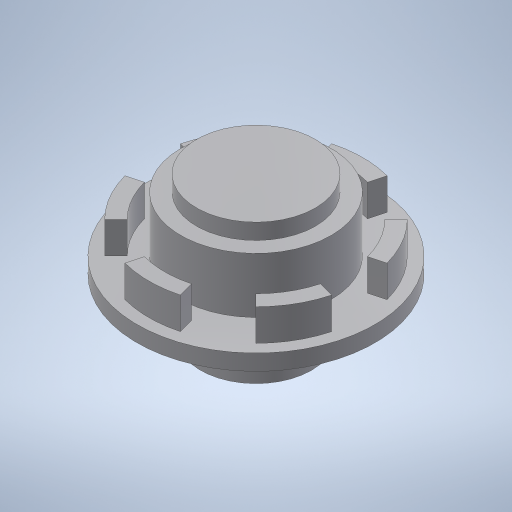
# Autodesk Inventor part: Bisagra final
Saved by Autodesk Inventor 2023.1 (Build 271208000, 208)
## iProperties
Created: 2022-10-06
Part Number: Bisagra final
Material: Generic
Document SubType Name: Modeling
Designer: User
Density: 1 g/cm^3
Appearance: Smooth - White
Author: User
Autodesk Inventor part; units mm, degrees
ref_plane "YZ Plane" through (0, 0, 0) normal (1, 0, 0) x (0, 1, 0)
ref_plane "XZ Plane" through (0, 0, 0) normal (0, 1, 0) x (-1, 0, 0)
ref_plane "XY Plane" through (0, 0, 0) normal (0, 0, 1) x (1, 0, 0)
sketch "Sketch1" plane through (0, 0, 0) normal (0, 1, 0) x (-1, 0, 0)
  circle A0 centre (0, 0) radius 15
  dimension "d0" = 30
  constraints: 1 centre point, 1 coincident
  measures "d0" diameter of A0
extrude "Extrusion1" add sketch "Sketch1" along normal blind 2
sketch "Sketch2" plane through (0, 2, 0) normal (0, 1, 0) x (1, 0, 0)
  circle A0 centre (0, 0) radius 15 projected
  circle A1 centre (0, 0) radius 13.5
  circle A2 centre (0, 0) radius 11.5
  line L0 (11.1081, 2.9764) -> (13.04, 3.4941)
  line L1 (0, 0) -> (13.5, 0) construction
  line L2 (11.1081, -2.9764) -> (13.04, -3.4941)
  line L3 (0, 0) -> (13.5, 0) construction
  line L4 (8.1317, 8.1317) -> (9.5459, 9.5459)
  line L5 (0, 0) -> (13.5, 0) construction
  line L6 (2.9764, 11.1081) -> (3.4941, 13.04)
  line L7 (0, 0) -> (13.5, 0) construction
  line L8 (-2.9764, 11.1081) -> (-3.4941, 13.04)
  circle A3 centre (0, 0) radius 15 projected
  line L9 (-8.1317, 8.1317) -> (-9.5459, 9.5459)
  line L10 (0, 0) -> (13.5, 0) construction
  line L11 (-9.5459, 9.5459) -> (-8.1317, 8.1317)
  line L12 (8.1317, -8.1317) -> (9.5459, -9.5459)
  line L13 (-3.4941, 13.04) -> (-2.9764, 11.1081)
  line L14 (2.9764, -11.1081) -> (3.4941, -13.04)
  line L15 (9.5459, 9.5459) -> (8.1317, 8.1317)
  line L16 (-8.1317, -8.1317) -> (-9.5459, -9.5459)
  line L17 (3.4941, 13.04) -> (2.9764, 11.1081)
  line L18 (-2.9764, -11.1081) -> (-3.4941, -13.04)
  line L19 (13.04, 3.4941) -> (11.1081, 2.9764)
  line L20 (-11.1081, -2.9764) -> (-13.04, -3.4941)
  line L21 (13.04, -3.4941) -> (11.1081, -2.9764)
  line L22 (-11.1081, 2.9764) -> (-13.04, 3.4941)
  constraints: 46 end point, 6 point on line, 5 horizontal, 2 perpendicular, 28 other
extrude "Extrusion2" add sketch "Sketch2" along normal blind 4 contours L0 A2 L4 A1 | A1 L12 A2 L2 | L6 A2 L8 A1 | A1 L18 A2 L14 | L9 A2 L22 A1 | A1 L20 A2 L16
sketch "Sketch3" plane through (0, 2, 0) normal (0, 1, 0) x (1, 0, 0)
  line L0 (-2.9764, 11.1081) -> (-3.4941, 13.04) projected
  arc A0 (3.4941, 13.04) -> (-3.4941, 13.04) centre (0, 0) ccw projected
  line L1 (3.4941, 13.04) -> (2.9764, 11.1081) projected
  arc A1 (2.9764, 11.1081) -> (-2.9764, 11.1081) centre (0, 0) ccw projected
  line L2 (-3.4941, -13.04) -> (-2.9764, -11.1081) projected
  arc A2 (-2.9764, -11.1081) -> (2.9764, -11.1081) centre (0, 0) ccw projected
  line L3 (2.9764, -11.1081) -> (3.4941, -13.04) projected
  arc A3 (-3.4941, -13.04) -> (3.4941, -13.04) centre (0, 0) ccw projected
  line L4 (-11.1081, 2.9764) -> (-13.04, 3.4941) projected
  arc A4 (-9.5459, 9.5459) -> (-13.04, 3.4941) centre (0, 0) ccw projected
  line L5 (-9.5459, 9.5459) -> (-8.1317, 8.1317) projected
  arc A5 (-8.1317, 8.1317) -> (-11.1081, 2.9764) centre (0, 0) ccw projected
  line L6 (8.1317, 8.1317) -> (9.5459, 9.5459) projected
  arc A6 (13.04, 3.4941) -> (9.5459, 9.5459) centre (0, 0) ccw projected
  line L7 (13.04, 3.4941) -> (11.1081, 2.9764) projected
  arc A7 (11.1081, 2.9764) -> (8.1317, 8.1317) centre (0, 0) ccw projected
  line L8 (9.5459, -9.5459) -> (8.1317, -8.1317) projected
  arc A8 (8.1317, -8.1317) -> (11.1081, -2.9764) centre (0, 0) ccw projected
  line L9 (11.1081, -2.9764) -> (13.04, -3.4941) projected
  arc A9 (9.5459, -9.5459) -> (13.04, -3.4941) centre (0, 0) ccw projected
  line L10 (-13.04, -3.4941) -> (-11.1081, -2.9764) projected
  arc A10 (-11.1081, -2.9764) -> (-8.1317, -8.1317) centre (0, 0) ccw projected
  line L11 (-8.1317, -8.1317) -> (-9.5459, -9.5459) projected
  arc A11 (-13.04, -3.4941) -> (-9.5459, -9.5459) centre (0, 0) ccw projected
  circle A12 centre (0, 0) radius 15 projected
  circle A13 centre (0, 0) radius 9.5
  dimension "d12" = 19
  constraints: 1 centre point, 1 coincident
  measures "d12" diameter of A13
extrude "Extrusion3" add sketch "Sketch3" along normal blind 7 contours A13
sketch "Sketch4" plane through (0, 9, 0) normal (0, 1, 0) x (1, 0, 0)
  circle A0 centre (0, 0) radius 9.5 projected
  circle A1 centre (0, 0) radius 7.5
  dimension "d15" = 15
  constraints: 1 centre point, 1 coincident
  measures "d15" diameter of A1
extrude "Extrusion4" add sketch "Sketch4" along normal blind 2 contours A1
sketch "Sketch5" plane through (0, 0, 0) normal (0, -1, 0) x (1, 0, 0)
  circle A0 centre (0, 0) radius 7
  dimension "d18" = 14
  constraints: 1 centre point, 1 coincident
  measures "d18" diameter of A0
extrude "Extrusion5" add sketch "Sketch5" along normal blind 7
body "Solid1"
